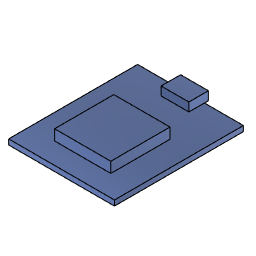
Macap digital (Autodesk Fusion 360 archive; units mm, degrees)
design "Wemos D1 Mini"
Autodesk Fusion 360 part; units mm, degrees
sketch "Sketch1" plane through (0, 0, 0) normal (0, 0, 1) x (1, 0, 0)
  line L0 (0, 0) -> (32, 0)
  line L1 (32, 0) -> (32, 39)
  line L2 (32, 39) -> (0, 39)
  line L3 (0, 39) -> (0, 0)
  dimension "d1" = 32
  dimension "d2" = 39
  constraint horizontal L0
  constraint vertical L1
  constraint horizontal L2
  constraint vertical L3
  constraint coincident L0.start L3.end
  measures "d1" distance of L0.start L0.end
  measures "d2" distance of L0.start L2.end
extrude "Extrude1" add sketch "Sketch1" along normal blind 1.6
sketch "Sketch2" plane through (0, 0, 1.6) normal (0, 0, 1) x (-1, 0, 0)
  line L0 (0, -39) -> (0, 0)
  line L1 (0, 0) -> (-32, 0)
  line L2 (-32, 0) -> (-32, -39)
  line L3 (-32, -39) -> (0, -39)
  line L4 (-7.5, -24.3) -> (-24.5, -24.3)
  line L5 (-24.5, -24.3) -> (-24.5, -6.4)
  line L6 (-24.5, -6.4) -> (-7.5, -6.4)
  line L7 (-7.5, -6.4) -> (-7.5, -24.3)
  dimension "d5" = 14.7
  dimension "d6" = 6.4
  dimension "d7" = 7.5
  dimension "d8" = 7.5
  constraint horizontal L4
  constraint vertical L5
  constraint horizontal L6
  constraint vertical L7
  measures "d5" distance of L3 L4
  measures "d6" distance of L1 L6
  measures "d7" distance of L0 L7
  measures "d8" distance of L2 L5
extrude "Extrude2" add sketch "Sketch2" along normal blind 3.2 contours L4 L5 L6 L7
sketch "Sketch3" plane through (0, 0, 1.6) normal (0, 0, 1) x (-1, 0, 0)
  line L0 (-7.5, -6.4) -> (-7.5, -24.3)
  line L1 (-7.5, -24.3) -> (-24.5, -24.3)
  line L2 (-24.5, -24.3) -> (-24.5, -6.4)
  line L3 (-24.5, -6.4) -> (-7.5, -6.4)
  line L4 (0, -39) -> (0, 0)
  line L5 (0, 0) -> (-32, 0)
  line L6 (-32, 0) -> (-32, -39)
  line L7 (-32, -39) -> (0, -39)
  line L8 (-11.8, -34.3) -> (-20.2, -34.3)
  line L9 (-20.2, -34.3) -> (-20.2, -40.2)
  line L10 (-20.2, -40.2) -> (-11.8, -40.2)
  line L11 (-11.8, -40.2) -> (-11.8, -34.3)
  dimension "d11" = 11.8
  dimension "d12" = 11.8
  dimension "d14" = 1.2
  dimension "d15" = 4.7
  constraint horizontal L8
  constraint vertical L9
  constraint horizontal L10
  constraint vertical L11
  measures "d11" distance of L6 L9
  measures "d12" distance of L4 L11
  measures "d14" distance of L7 L10
  measures "d15" distance of L7 L8
extrude "Extrude3" add sketch "Sketch3" along normal blind 2.6 contours L7 L9 L10 L11 | L7 L8 L9 L11
equation "d9 = 4.8 mm - 1.6 mm"
equation "d16 = 4.2 mm - 1.6 mm"
